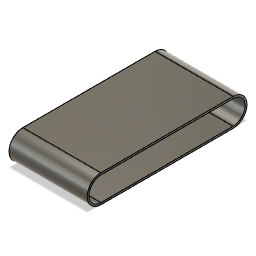
Конвейерная лента v2 (Autodesk Fusion 360 design; units mm, degrees)
Autodesk Fusion 360 part; units mm, degrees
sketch "Sketch1" plane through (0, 0, 0) normal (1, 0, 0) x (0, 0, -1)
  line L0 (-220, 20) -> (0, 20)
  line L1 (0, -20) -> (-220, -20)
  arc A0 (-220, 20) -> (-220, -20) centre (-220, 0) ccw
  arc A1 (0, -20) -> (0, 20) centre (0, 0) ccw
  arc A2 (0, -23) -> (0, 23) centre (0, 0) ccw
  line L2 (-220, 23) -> (0, 23)
  arc A3 (-220, 23) -> (-220, -23) centre (-220, 0) ccw
  line L3 (0, -23) -> (-220, -23)
  dimension "d2" = 40
  dimension "d3" = 40
  dimension "d4" = 220
  dimension "d5" = 220
  dimension "d6" = 220
  dimension "d7" = -3
  constraint coincident A1.centre A2.centre
  constraint tangent L0 A1
  constraint horizontal L0
  constraint tangent L1 A0
  measures "d2" diameter of A0
  measures "d3" diameter of A1
  measures "d4" distance of L0.start L0.end
  measures "d5" distance of L1.start L1.end
  measures "d6" distance of A1.centre A0.centre
extrude "Extrude1" add sketch "Sketch1" along normal blind 130
